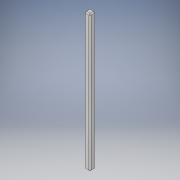
# Autodesk Inventor part: frame
Saved by Autodesk Inventor 2019 (Build 230136000, 136)
## iProperties
Created: 2020-02-11
Part Number: frame
Material: Generic
Document SubType Name: Modeling
Designer: Vinayak
Density: 1 g/cm^3
Appearance: Default
Author: Vinayak
Autodesk Inventor part; units mm, degrees
ref_plane "YZ Plane" through (0, 0, 0) normal (1, 0, 0) x (0, 1, 0)
ref_plane "XZ Plane" through (0, 0, 0) normal (0, 1, 0) x (-1, 0, 0)
ref_plane "XY Plane" through (0, 0, 0) normal (0, 0, 1) x (1, 0, 0)
sketch "Sketch1" plane through (0, 0, 0) normal (0, 0, 1) x (1, 0, 0)
  line L0 (0, 0) -> (25, 0)
  line L1 (25, 0) -> (25, 600)
  line L2 (25, 600) -> (0, 600)
  line L3 (0, 600) -> (0, 0)
  dimension "d0" = 25
  dimension "d1" = 600
  constraints: 8 end point, 2 parallel, 1 horizontal, 1 perpendicular
  measures "d0" distance of L2.end L1.end
  measures "d1" distance of L1.end L0.end
extrude "Extrusion1" add sketch "Sketch1" along normal blind 25
chamfer "Chamfer1" distance 5 angle 45 12 edges at (25, 300, 25) (25, 300, 0) (0, 300, 25) (0, 600, 12.5) (12.5, 600, 0) (12.5, 600, 25) (25, 600, 12.5) (25, 0, 12.5) (12.5, 0, 25) (12.5, 0, 0) (0, 0, 12.5) (0, 300, 0)
body "Solid1"
